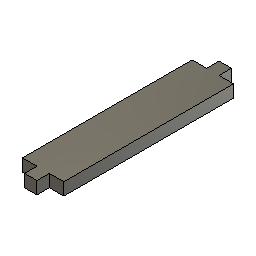
Akkuhalterung v1 (Autodesk Fusion 360 design; units mm, degrees)
Autodesk Fusion 360 part; units mm, degrees
sketch "Skizze1" plane through (0, 0, 0) normal (0, 1, 0) x (1, 0, 0)
  line L0 (0, 0) -> (3, 0)
  line L1 (3, 0) -> (3, 3)
  line L2 (0, 0) -> (0, 3)
  line L3 (3, 3) -> (6.5, 3)
  line L4 (6.5, 3) -> (6.5, 3.4599)
  line L5 (0, 3) -> (-3.5, 3)
  line L6 (1.5, 0) -> (1.5, 47)
  line L7 (1.5, 47) -> (3, 47)
  line L8 (3, 47) -> (0, 47)
  line L9 (0, 47) -> (0, 44)
  line L10 (3, 47) -> (3, 44)
  line L11 (6.5, 3) -> (6.5, 44)
  line L12 (6.5, 44) -> (3, 44)
  line L13 (-3.5, 3) -> (-3.5, 44)
  line L14 (-3.5, 44) -> (0, 44)
  dimension "d1" = 3
  dimension "d2" = 3
  dimension "d3" = 3
  dimension "d4" = 3.5
  dimension "d5" = 3.5
  dimension "d6" = 47
  dimension "d7" = 1.5
  dimension "d8" = 3
  dimension "d9" = 3
  constraint coincident L0.start L2.start
  constraint horizontal L0
  constraint perpendicular L0 L1
  constraint perpendicular L0 L2
  constraint perpendicular L1 L3
  constraint perpendicular L3 L4
  constraint perpendicular L2 L5
  constraint midpoint L0 L6.start
  constraint perpendicular L0 L6
  constraint perpendicular L6 L7
  constraint perpendicular L6 L8
  constraint perpendicular L8 L9
  constraint perpendicular L8 L10
  constraint perpendicular L3 L11
  constraint perpendicular L10 L12
  constraint perpendicular L5 L13
  constraint perpendicular L9 L14
  measures "d1" distance of L0.start L0.end
  measures "d2" distance of L0.end L1.end
  measures "d3" distance of L0.start L2.end
  measures "d4" distance of L1.end L3.end
  measures "d5" distance of L2.end L5.end
  measures "d6" distance of L6.start L6.end
  measures "d7" distance of L6.end L7.end
  measures "d8" distance of L8.end L9.end
  measures "d9" distance of L7.end L10.end
extrude "Extrusion1" add sketch "Skizze1" along normal blind 3
